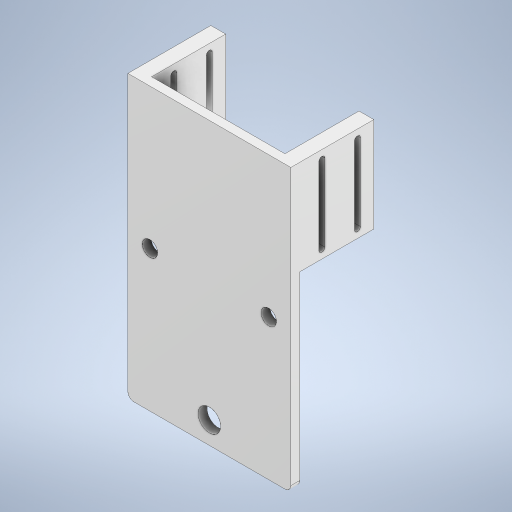
# Autodesk Inventor part: Electromagnet Gantry Plate
Saved by Autodesk Inventor 2023.2 (Build 272271030, 271C)
## iProperties
Created: 2023-04-10
Part Number: Electromagnet Gantry Plate
Material: PC/ABS Plastic
Document SubType Name: Modeling
Designer: ethan
Density: 0.357273 g/cm^3
Appearance: Smooth - White
Author: ethan
Autodesk Inventor part; units mm, degrees
ref_plane "YZ Plane" through (0, 0, 0) normal (1, 0, 0) x (0, 1, 0)
ref_plane "XZ Plane" through (0, 0, 0) normal (0, 1, 0) x (-1, 0, 0)
ref_plane "XY Plane" through (0, 0, 0) normal (0, 0, 1) x (1, 0, 0)
sketch "Sketch1" plane through (0, 0, 0) normal (0, 1, 0) x (-1, 0, 0)
  line L0 (0, 0) -> (55, 0)
  line L1 (55, 0) -> (55, -55)
  line L2 (55, -55) -> (0, -55)
  line L3 (0, -55) -> (0, 0)
  line L4 (47.55, -7.45) -> (7.45, -7.45) construction
  line L5 (7.45, -7.45) -> (7.45, -47.55) construction
  line L6 (7.45, -47.55) -> (47.55, -47.55) construction
  line L7 (47.55, -47.55) -> (47.55, -7.45) construction
  circle A0 centre (47.55, -7.45) radius 2.6
  circle A1 centre (47.55, -47.55) radius 2.6
  circle A2 centre (7.45, -47.55) radius 2.6
  circle A3 centre (7.45, -7.45) radius 2.6
  circle A4 centre (47.55, -7.45) radius 12.5 construction
  circle A5 centre (27.5, -7.45) radius 3.8
  dimension "d0" = 55
  dimension "d1" = 55
  dimension "d2" = 40.1
  dimension "d3" = 40.1
  dimension "d4" = 5.2
  dimension "d5" = 5.2
  dimension "d6" = 5.2
  dimension "d7" = 5.2
  dimension "d8" = 7.45
  dimension "d9" = 7.45
  dimension "d13" = 25
  dimension "d78" = 7.6
  constraints: 16 end point, 6 centre point, 5 coincident, 4 parallel, 2 horizontal, 2 perpendicular, 1 midpoint
  measures "d0" distance of L1.end L2.end
  measures "d1" distance of L0.end L1.end
  measures "d2" distance of L6.end L5.end
  measures "d3" distance of L5.end L4.end
  measures "d4" diameter of A0
  measures "d5" diameter of A3
  measures "d6" diameter of A1
  measures "d7" diameter of A2
  measures "d8" distance between parallel lines of L1 L7
  measures "d9" distance from line of L2 L5.end
  measures "d13" diameter of A4
  measures "d78" diameter of A5
extrude "Extrusion1" add sketch "Sketch1" along normal blind 3 contours L0 L1 L2 L3 | A0 | A3
fillet "Fillet1" radius 2 2 edges at (-55, 1.5, 0) (0, 1.5, 0)
sketch "Sketch3" plane through (0, 0, -53) normal (1, 0, 0) x (0, 0, -1)
  line L0 (-13, 0) -> (-13, -20) construction
  line L1 (12, -20) -> (-13, -20) construction
  line L2 (-13, 0) -> (-33, 0) construction
  line L3 (-33, 0) -> (-33, -20) construction
  line L4 (-33, -20) -> (-13, -20) construction
  line L5 (-13, -20) -> (-13, 0) construction
  line L6 (2, 0) -> (-13, 0) construction
  line L7 (-13, 0) -> (-33, -20) construction
  line L8 (-33, -10) -> (-13, -10) projected
  circle A0 centre (-23, -10) radius 5
  point P0 (-53, 0)
  point P1 (2, -20)
  dimension "d25" = 10
  constraints: 10 end point, 2 parallel, 1 centre point, 1 horizontal, 1 midpoint, 1 perpendicular
  measures "d25" diameter of A0
extrude "Extrusion3" cut sketch "Sketch3" against normal blind 12
sketch "Sketch4" plane through (-55, 0, -2) normal (-1, 0, 0) x (0, 0, 1)
  circle A0 centre (-28, -10) radius 5 projected
  circle A1 centre (-28, -10) radius 2.75
  point P0 (2, 0)
  dimension "d30" = 5.5
  constraints: 1 centre point, 1 coincident
  measures "d30" diameter of A1
extrude "Extrusion4" cut sketch "Sketch4" against normal blind 12 contours A0 | A1
extrude "Extrusion5" cut sketch "Sketch4" against normal through all contours A1
sketch "Sketch5" plane through (-53, 3, 0) normal (0, 0, 1) x (1, 0, 0)
  line L0 (35.5, -3) -> (35.5, -23) construction
  line L1 (15.5, -3) -> (15.5, -23) construction
  line L2 (35.5, -3) -> (15.5, -3) construction
  line L3 (15.5, -3) -> (15.5, -23) construction
  line L4 (15.5, -23) -> (35.5, -23) construction
  line L5 (35.5, -23) -> (35.5, -3) construction
  line L6 (15.5, -23) -> (35.5, -23) construction
  line L7 (15.5, -3) -> (-2, -3) construction
  line L8 (35.5, -23) -> (15.5, -3) construction
  circle A0 centre (25.5, -13) radius 5
  circle A1 centre (25.5, -13) radius 2.75
  point P0 (53, -3)
  dimension "d33" = 10
  dimension "d34" = 5.5
  constraints: 10 end point, 2 centre point, 2 parallel, 1 coincident, 1 horizontal, 1 midpoint, 1 perpendicular
  measures "d33" diameter of A0
  measures "d34" diameter of A1
extrude "Extrusion6" cut sketch "Sketch5" against normal blind 12 contours A0 | A1
ref_plane "Work Plane1" through (0, 0, 0) normal (0, 1, 0) x (1, 0, 0)
sketch "Sketch7" plane through (0, 0, 0) normal (0, 1, 0) x (1, 0, 0)
  line L0 (-19.45, 63) -> (-19.45, 53.4092)
  line L1 (-35.55, 19.45) -> (-35.55, 63) projected
  line L2 (-19.45, 55) -> (-35.55, 55)
  line L3 (-35.55, 55) -> (-35.55, 63)
  line L4 (-35.55, 63) -> (-19.45, 63)
  line L5 (-19.45, 63) -> (-19.45, 55)
  circle A0 centre (-47.55, 47.55) radius 2.6 projected
  circle A1 centre (-47.55, 47.55) radius 12
  circle A2 centre (-7.45, 47.55) radius 2.6 projected
  circle A3 centre (-7.45, 47.55) radius 12
  point P0 (0, 0)
  point P1 (-53, 55)
  dimension "d67" = 24
  dimension "d68" = 24
  constraints: 10 end point, 2 centre point, 2 coincident, 2 parallel, 1 horizontal, 1 perpendicular, 1 point on line
  measures "d67" diameter of A1
  measures "d68" diameter of A3
extrude "Extrusion9" add sketch "Sketch7" along normal blind 25 contours L0 L2 L1 L4
ref_plane "Work Plane3" through (-19.45, -5, -63) normal (0, 0, -1) x (-1, 0, 0)
ref_plane "Work Plane2" through (-19.45, -5, -63) normal (0, 0, -1) x (-1, 0, 0)
sketch "Sketch9" plane through (-19.45, -5, -63) normal (0, 0, -1) x (-1, 0, 0)
  line L0 (0, 0) -> (0, 8) projected
  line L1 (16.1, 8) -> (16.1, 5) projected
  line L2 (0, 8) -> (16.1, 8)
  line L3 (4.55, 8) -> (11.55, 8) projected
  line L4 (8.05, 8) -> (8.05, 21.475)
  circle A0 centre (8.05, 21.475) radius 3
  point P0 (-19.45, 5)
  dimension "d54" = 13.475
  dimension "d55" = 6
  constraints: 4 end point, 1 centre point, 1 coincident, 1 midpoint, 1 perpendicular, 1 vertical
  measures "d54" distance of L4.start L4.end
  measures "d55" diameter of A0
extrude "Extrusion11" cut sketch "Sketch9" against normal through all
sketch "Sketch10" plane through (-19.45, 0, -63) normal (0, 0, -1) x (-1, 0, 0)
  circle A0 centre (8.05, 16.475) radius 3 projected
  arc A1 (23.05, 16.475) -> (-6.95, 16.475) centre (8.05, 16.475) ccw
  line L0 (-6.95, 16.475) -> (-6.95, 0)
  line L1 (23.05, 16.475) -> (23.05, 0)
  line L2 (-6.95, 0) -> (23.05, 0)
  line L3 (33.55, 0) -> (-17.45, 0) projected
  point P0 (-19.45, 0)
  dimension "d60" = 30
  constraints: 6 end point, 2 point on circle, 2 tangent, 2 vertical, 1 centre point, 1 coincident, 1 collinear
  measures "d60" diameter of A1
extrude "Extrusion12" add sketch "Sketch10" against normal up to surface (8 mm away)
chamfer "Chamfer2" distance 6.75 angle 45 1 edges at (-27.5, 31.475, -55)
sketch "Sketch11" plane through (0, 0, 0) normal (0, -1, 0) x (1, 0, 0)
  line L0 (0, -2) -> (0, -55) projected
  line L1 (-19.45, -63) -> (0, -63)
  line L2 (0, -63) -> (0, -55)
  line L3 (0, -55) -> (-19.45, -55)
  line L4 (-19.45, -55) -> (-19.45, -63)
  line L5 (-19.45, -63) -> (-35.55, -63) projected
  line L6 (-55, -55) -> (-55, -2) projected
  line L7 (-35.55, -63) -> (-55, -63)
  line L8 (-55, -63) -> (-55, -55)
  line L9 (-55, -55) -> (-35.55, -55)
  line L10 (-35.55, -55) -> (-35.55, -63)
  point P0 (0, 0)
  constraints: 16 end point, 4 parallel, 2 horizontal, 2 perpendicular
extrude "Extrusion13" add sketch "Sketch11" against normal up to surface (3 mm away)
sketch "Sketch13" plane through (0, 0, 0) normal (0, -1, 0) x (1, 0, 0)
  line L0 (0, -2) -> (0, -63) projected
  line L1 (0, -63) -> (-55, -63)
  line L2 (-55, -63) -> (-55, -83)
  line L3 (-55, -83) -> (0, -83)
  line L4 (0, -83) -> (0, -63)
  point P0 (0, 0)
  dimension "d79" = 20
  constraints: 8 end point, 2 parallel, 1 horizontal, 1 perpendicular
  measures "d79" distance of L2.end L1.end
extrude "Extrusion15" add sketch "Sketch13" against normal up to surface (3 mm away)
sketch "Sketch14" plane through (0, 3, 0) normal (0, 1, 0) x (1, 0, 0)
  line L0 (0, 2) -> (0, 83) projected
  line L1 (0, 80.6806) -> (0, 63)
  line L2 (0, 63) -> (-55, 63)
  line L3 (0, 63) -> (0, 95)
  line L4 (0, 95) -> (-55, 95)
  line L5 (-55, 63) -> (-55, 95)
  point P0 (0, 0)
  dimension "d93" = 32
  constraints: 10 end point, 2 point on line, 1 horizontal, 1 perpendicular
  measures "d93" distance of L1.end L3.end
extrude "Extrusion16" add sketch "Sketch14" along normal blind 25 and the other way blind 3
sketch "Sketch16" plane through (-55, 0, -2) normal (-1, 0, 0) x (0, 0, 1)
  line L0 (-53, 19.475) -> (-53, 13.475) projected
  line L1 (-90, 21.475) -> (-64, 21.475)
  line L2 (-64, 23.475) -> (-90, 23.475)
  arc A0 (-90, 23.475) -> (-90, 21.475) centre (-90, 22.475) ccw
  arc A1 (-64, 21.475) -> (-64, 23.475) centre (-64, 22.475) ccw
  line L3 (-93, 28) -> (-93, 0) projected
  line L4 (-61, 28) -> (-93, 28) projected
  line L5 (0, 0) -> (-93, 0) projected
  line L6 (-90, 9.475) -> (-64, 9.475)
  line L7 (-64, 11.475) -> (-90, 11.475)
  arc A2 (-90, 11.475) -> (-90, 9.475) centre (-90, 10.475) ccw
  arc A3 (-64, 9.475) -> (-64, 11.475) centre (-64, 10.475) ccw
  point P0 (2, 0)
  point P1 (-49.4408, 16.475)
  constraints: 8 end point, 8 point on circle, 8 tangent, 4 centre point, 2 parallel
sketch "Sketch17" plane through (0, 28, -95) normal (0, 0, -1) x (-1, 0, 0)
  arc A0 (37.1007, 0) -> (17.8993, 0) centre (27.5, -11.525) ccw projected
  line L0 (44.95, -28) -> (50.15, -28) projected
  line L1 (46.5, -28) -> (8.5, -28)
  line L2 (5, 0) -> (50, 0)
  line L3 (55, -28) -> (0, -28)
  line L4 (50, -25) -> (5, -25)
  line L5 (50, 0) -> (50, -25)
  line L6 (27.75, -25) -> (27.25, -25) projected
  arc A1 (35.75, -11.525) -> (19.25, -11.525) centre (27.5, -11.525) ccw projected
  line L7 (27.5, -25) -> (27.5, -11.525)
  line L8 (5, 0) -> (5, -25)
  point P0 (55, 0)
  point P1 (40.8949, -25)
  point P2 (50, -28)
  point P3 (39.8, -25)
  point P4 (15.2, -25)
  point P5 (35.55, -13.3305)
  point P6 (19.45, -13.3305)
  point P7 (5, -28)
  dimension "d97" = 3
  constraints: 14 end point, 3 point on line, 2 parallel, 2 symmetric about line, 1 collinear, 1 horizontal, 1 midpoint, 1 perpendicular, 1 vertical
  measures "d97" distance between parallel lines of L1 L4
extrude "Extrusion18" cut sketch "Sketch17" against normal up to surface (32 mm away) contours L2 L5 L4 L8
extrude "Extrusion19" cut sketch "Sketch16" against normal through all
fillet "Fillet9" radius 12.75 3 edges at (-39.125, 3, -58.375) (-27.5, 3, -55) (-15.875, 3, -58.375)
equation "\"d1\" = d0"
equation "\"d3\" = d2"
equation "\"d5\" = d4"
equation "\"d6\" = d4"
equation "\"d7\" = d4"
equation "\"d8\" = -0.5 * d2 + 0.5 * d0"
equation "\"d9\" = -0.5 * d3 + 0.5 * d1"
body "Solid1"
